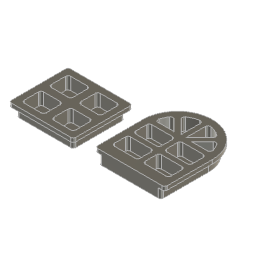
gingerbread-house (Autodesk Fusion 360 design; units mm, degrees)
Autodesk Fusion 360 part; units mm, degrees
note: some values were not read from the file. Set by a fixed rule: which sketch regions a step uses.
sketch "base" plane through (0, 0, 0) normal (0, 0, 1) x (1, 0, 0)
  line L0 (0, 0) -> (22, 0)
  line L1 (22, 0) -> (22, 20)
  line L2 (22, 20) -> (0, 20)
  line L3 (0, 20) -> (0, 0)
  line L4 (32, 0) -> (56, 0)
  line L5 (56, 0) -> (56, 18.5)
  line L6 (32, 18.5) -> (32, 0)
  line L7 (32, 18.5) -> (56, 18.5) construction
  arc A0 (56, 18.5) -> (32, 18.5) centre (44, 18.5) ccw
  dimension "d1" = 22
  dimension "d2" = 20
  dimension "d20" = 24
  dimension "d21" = 18.5
  dimension "d22" = 10
  constraint horizontal L0
  constraint vertical L1
  constraint horizontal L2
  constraint vertical L3
  constraint coincident L0.start L3.end
  constraint horizontal L4
  constraint vertical L5
  constraint vertical L6
  constraint collinear L0 L4
  constraint perpendicular L5 L7
  constraint midpoint L7 A0.centre
  measures "d1" distance of L0.start L0.end
  measures "d2" distance of L0.start L2.end
  measures "d20" distance of L4.start L4.end
  measures "d21" distance of L4.start L6.start
  measures "d22" distance of L0.end L4.start
extrude "insert" add sketch "base" along normal blind 3.5 makes body 1 at (7.3333, 13.3333, 0) makes body 2 at (48, 12.3333, 0)
sketch "upper" plane through (0, 0, 3.5) normal (0, 0, 1) x (-1, 0, 0)
  line L0 (-32, -18.5) -> (-32, 0) construction
  line L1 (-56, 0) -> (-56, -18.5) construction
  line L2 (-32, 0) -> (-56, 0) construction
  line L3 (-57.5, 0) -> (-57.5, -18.5)
  line L4 (-30.5, -18.5) -> (-30.5, 0)
  line L5 (-30.5, 0) -> (-57.5, 0)
  arc A0 (-56, -18.5) -> (-32, -18.5) centre (-44, -18.5) ccw construction
  line L6 (-32, -18.5) -> (-32, 0) construction
  line L7 (-32, 0) -> (-56, 0)
  line L8 (-56, 0) -> (-56, -18.5) construction
  arc A1 (-57.5, -18.5) -> (-30.5, -18.5) centre (-44, -18.5) ccw
  line L9 (-44, -18.5) -> (-57.5, -18.5) construction
  line L10 (-44, -18.5) -> (-30.5, -18.5) construction
  line L11 (-44, -18.5) -> (-30.5, -18.5) construction
  line L12 (-22, -20) -> (0, -20) construction
  line L13 (0, -20) -> (0, 0) construction
  line L14 (0, 0) -> (-22, 0) construction
  line L15 (-22, 0) -> (-22, -20) construction
  line L16 (1.5, 1.5) -> (-23.5, 1.5)
  line L17 (-23.5, 1.5) -> (-23.5, -21.5)
  line L18 (-23.5, -21.5) -> (1.5, -21.5)
  line L19 (1.5, -21.5) -> (1.5, 1.5)
  dimension "d58" = 180
  dimension "d62" = 1.5
  dimension "d76" = 1.5
  constraint perpendicular L3 L5
  constraint collinear L2 L5
  constraint coincident A0.centre A1.centre
  constraint perpendicular L0 L11
  constraint coincident L4.start A1.end
  measures "d58" angle of L9 L10
  measures "d76" distance of L0 L4
extrude "main" add sketch "upper" along normal blind 1.5 bodies 1 2
sketch "face" plane through (0, 0, 5) normal (0, 0, 1) x (-1, 0, 0)
  line L0 (-11, -21.5) -> (-11, 1.5) construction
  line L1 (1.5, -10) -> (-23.5, -10) construction
  line L2 (-32, 0) -> (-56, 0)
  line L3 (-32, -18.5) -> (-32, 0)
  arc A0 (-55, -18.5) -> (-33, -18.5) centre (-44, -18.5) ccw
  line L4 (-55, -18.5) -> (-55, -4)
  line L5 (-55, -4) -> (-33, -4)
  line L6 (-33, -4) -> (-33, -18.5)
  line L7 (-33, -11.25) -> (-55, -11.25) construction
  line L8 (-44, -4) -> (-44, -29.5) construction
  line L9 (-33, -18.5) -> (-55, -18.5) construction
  line L10 (-44, -18.5) -> (-51.7782, -26.2782) construction
  line L11 (-44, -18.5) -> (-36.2218, -26.2782) construction
  line L12 (-44, -18.5) -> (-33, -18.5) construction
  line L13 (-45, -20.9142) -> (-51.0389, -26.9531)
  line L14 (-43, -20.9142) -> (-36.9611, -26.9531)
  line L15 (-33, -10.25) -> (-55, -10.25)
  line L16 (-33, -12.25) -> (-55, -12.25)
  line L17 (-33, -18.5) -> (-55, -18.5)
  line L18 (-43, -4) -> (-43, -18.5)
  line L19 (-43, -20.9142) -> (-43, -29.4545)
  line L20 (-45, -4) -> (-45, -19.5)
  line L21 (-45, -20.9142) -> (-45, -29.4545)
  line L22 (-33.1833, -20.5) -> (-40.5858, -20.5)
  line L23 (-47.4142, -20.5) -> (-54.8167, -20.5)
  line L24 (-40.5858, -20.5) -> (-35.5469, -25.5389)
  line L25 (-47.4142, -20.5) -> (-52.4531, -25.5389)
  line L26 (-56, 0) -> (-56, -18.5)
  arc A1 (-57.5, -18.5) -> (-30.5, -18.5) centre (-44, -18.5) ccw
  line L27 (-30.5, -18.5) -> (-30.5, 0)
  line L28 (-30.5, 0) -> (-57.5, 0)
  line L29 (-57.5, 0) -> (-57.5, -18.5)
  arc A2 (-56, -18.5) -> (-32, -18.5) centre (-44, -18.5) ccw
  arc A3 (-57.5, -18.5) -> (-30.5, -18.5) centre (-44, -18.5) ccw
  line L30 (-30.5, -18.5) -> (-30.5, 0)
  line L31 (-30.5, 0) -> (-57.5, 0)
  line L32 (-57.5, 0) -> (-57.5, -18.5)
  line L33 (1.5, -21.5) -> (1.5, 1.5)
  line L34 (1.5, 1.5) -> (-23.5, 1.5)
  line L35 (-23.5, 1.5) -> (-23.5, -21.5)
  line L36 (-23.5, -21.5) -> (1.5, -21.5)
  line L37 (-1, -19) -> (-9.5, -19)
  line L38 (-9.5, -19) -> (-9.5, -11.5)
  line L39 (-9.5, -11.5) -> (-1, -11.5)
  line L40 (-1, -11.5) -> (-1, -19)
  line L41 (-1, -1) -> (-9.5, -1)
  line L42 (-1, -8.5) -> (-1, -1)
  line L43 (-9.5, -8.5) -> (-1, -8.5)
  line L44 (-9.5, -1) -> (-9.5, -8.5)
  line L45 (-21, -19) -> (-12.5, -19)
  line L46 (-21, -11.5) -> (-21, -19)
  line L47 (-12.5, -11.5) -> (-21, -11.5)
  line L48 (-12.5, -19) -> (-12.5, -11.5)
  line L49 (-12.5, -1) -> (-12.5, -8.5)
  line L50 (-12.5, -8.5) -> (-21, -8.5)
  line L51 (-21, -8.5) -> (-21, -1)
  line L52 (-21, -1) -> (-12.5, -1)
  dimension "d29" = 45
  dimension "d36" = 1
  dimension "d37" = -1
  dimension "d40" = 4
  dimension "d41" = 1
  dimension "d42" = 1
  dimension "d60" = 45
  dimension "d67" = 2.5
  dimension "d68" = 2.5
  dimension "d69" = 3
  dimension "d70" = 3
  dimension "d71" = 1
  constraint tangent A0 L4
  constraint vertical L4
  constraint perpendicular L4 L5
  constraint vertical L6
  constraint midpoint L6 L7.start
  constraint midpoint L4 L7.end
  constraint midpoint L5 L8.start
  constraint midpoint A0 L8.end
  constraint perpendicular L5 L8
  constraint horizontal L12
  constraint coincident A0.centre L10.start
  constraint coincident A0 L14.end
  constraint coincident A0 L24.end
  constraint coincident A0 L11.end
  constraint coincident A0 L10.end
  constraint coincident A0 L13.end
  constraint coincident A0 L25.end
  constraint coincident A0 L23.end
  constraint coincident A0 L22.start
  constraint coincident L6 L16.start
  constraint coincident L6 L15.start
  constraint coincident L4 L16.end
  constraint coincident L4 L15.end
  constraint coincident A0 L6.end
  constraint coincident A0 L19.end
  constraint coincident A0 L21.end
  constraint collinear L18 L19
  constraint coincident L13.start L20
  constraint coincident L10 L20.end
  constraint collinear L20 L21
  constraint collinear L22 L23
  constraint coincident L9 L18.end
  constraint coincident L5 L18.start
  constraint coincident L5 L20.start
  constraint horizontal L37
  constraint vertical L38
  constraint horizontal L39
  constraint vertical L40
  constraint symmetric L1 L37.start L41.start
  constraint symmetric L1 L37.end L41.end
  constraint symmetric L1 L38.end L43.start
  constraint symmetric L1 L39.end L42.start
  constraint midpoint L1.start L33
  constraint midpoint L1.end L35
  constraint midpoint L0.start L36
  constraint midpoint L0.end L34
  constraint symmetric L0 L37.start L45.start
  constraint symmetric L0 L37.end L45.end
  constraint symmetric L0 L38.end L47.start
  constraint symmetric L0 L39.end L46.start
  constraint symmetric L0 L41.start L51.end
  constraint symmetric L0 L41.end L49.start
  constraint symmetric L0 L42.start L50.end
  constraint symmetric L0 L43.start L49.end
  measures "d29" angle of L11 L12
  measures "d40" distance of L2 L5
  measures "d41" distance of L11 L24
  measures "d42" distance of L10 L25
  measures "d60" angle of L9 L10
  measures "d67" distance of L33 L40
  measures "d68" distance of L36 L37
  measures "d69" distance of L39 L43
  measures "d70" distance of L38 L48
  measures "d71" distance of L3 L6
extrude "panes" cut sketch "face" against normal up to surface (4.8 mm away) contours L4 L16 L17 L20 | A0 L23 L25 | L4 L5 L15 L20 | L6 L16 L17 L18 | A0 L13 L21 | L5 L6 L15 L18 | A0 L22 L24 | A0 L14 L19 | L37 L38 L39 L40 | L41 L42 L43 L44 | L45 L46 L47 L48 | L49 L50 L51 L52 bodies 1 2
fillet "fillets" radius 1 52 edges at (1, 19, 2.6) (1, 11.5, 2.6) (1, 8.5, 2.6) (1, 1, 2.6) (9.5, 1, 2.6) (9.5, 8.5, 2.6) (9.5, 19, 2.6) (9.5, 11.5, 2.6) (12.5, 8.5, 2.6) (12.5, 1, 2.6) (21, 1, 2.6) (21, 19, 2.6) (21, 8.5, 2.6) (12.5, 19, 2.6) (12.5, 11.5, 2.6) (21, 11.5, 2.6) (-1.5, -1.5, 4.25) (23.5, -1.5, 4.25) (23.5, 21.5, 4.25) (-1.5, 21.5, 4.25) (0, 0, 1.75) (22, 0, 1.75) (0, 20, 1.75) (22, 20, 1.75) (35.5469, 25.5389, 2.6) (33.1833, 20.5, 2.6) (36.9611, 26.9531, 2.6) (43, 29.4545, 2.6) (45, 29.4545, 2.6) (51.0389, 26.9531, 2.6) (52.4531, 25.5389, 2.6) (54.8167, 20.5, 2.6) (33, 18.5, 2.6) (33, 12.25, 2.6) (33, 10.25, 2.6) (33, 4, 2.6) (43, 10.25, 2.6) (43, 4, 2.6) (43, 18.5, 2.6) (43, 12.25, 2.6) (45, 18.5, 2.6) (45, 12.25, 2.6) (45, 10.25, 2.6) (45, 4, 2.6) (55, 4, 2.6) (55, 10.25, 2.6) (55, 12.25, 2.6) (55, 18.5, 2.6) (56, 0, 1.75) (32, 0, 1.75) (30.5, 0, 4.25) (57.5, 0, 4.25) on bodies 1 2
equation "d37 = -d36"
named bodies: "window", "door"
